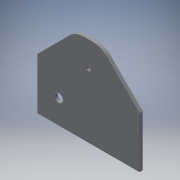
# Autodesk Inventor part: side Plate
Saved by Autodesk Inventor 2016 (Build 200138000, 138)
## iProperties
Created: 2016-11-04
Part Number: side Plate
Material: Generic
Document SubType Name: Modeling
Designer: william
Density: 1 g/cm^3
Appearance: Default
Author: william
Autodesk Inventor part; units mm, degrees
ref_plane "YZ Plane" through (0, 0, 0) normal (1, 0, 0) x (0, 1, 0)
ref_plane "XZ Plane" through (0, 0, 0) normal (0, 1, 0) x (-1, 0, 0)
ref_plane "XY Plane" through (0, 0, 0) normal (0, 0, 1) x (1, 0, 0)
sketch "Sketch1" plane through (0, 0, 0) normal (0, 1, 0) x (-1, 0, 0)
  line L0 (0, 0) -> (-200, 0)
  line L1 (-200, 0) -> (-200, 100)
  line L2 (-108.4315, 175) -> (-91.5685, 175)
  line L3 (0, 100) -> (0, 0)
  line L4 (0, 100) -> (-63.2843, 163.2843)
  line L5 (-200, 100) -> (-136.7157, 163.2843)
  arc A0 (-63.2843, 163.2843) -> (-91.5685, 175) centre (-91.5685, 135) ccw
  arc A1 (-108.4315, 175) -> (-136.7157, 163.2843) centre (-108.4315, 135) ccw
  circle A2 centre (-100, 125) radius 4
  point P0 (-75, 175)
  point P1 (-125, 175)
  point P2 (-100, 175)
  dimension "d0" = 200
  dimension "d1" = 100
  dimension "d2" = 135
  dimension "d3" = 135
  dimension "d4" = 50
  dimension "d5" = 40
  dimension "d8" = 8
  dimension "d9" = 50
  constraints: 12 end point, 4 point on circle, 4 point on line, 4 tangent, 3 centre point, 3 parallel, 1 equal radius, 1 horizontal, 1 midpoint, 1 perpendicular, 1 vertical alignment
  measures "d0" distance of L0.start L0.end
  measures "d1" distance of L0.end L1.end
  measures "d2" angle of L3 L4
  measures "d3" angle of L1 L5
  measures "d4" distance of point (-125, 175) point (-75, 175)
  measures "d5" radius of A0
  measures "d8" diameter of A2
  measures "d9" distance from line of L2 A2.centre
extrude "Extrusion1" add sketch "Sketch1" along normal blind 6.35
sketch "Sketch2" plane through (0, 0, 0) normal (0, -1, 0) x (1, 0, 0)
  circle A0 centre (41.967, 46.6929) radius 8.3401
  point P0 (0, 0)
  constraints: 1 centre point
extrude "Extrusion2" cut sketch "Sketch2" against normal blind 10
body "Solid1"
